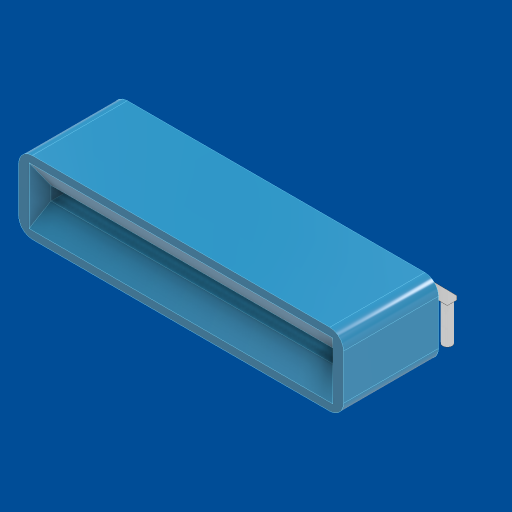
# Autodesk Inventor part: EEC12DRAN
Saved by Autodesk Inventor 2023.2 (Build 272271000, 271)
## iProperties
Created: 2023-01-27
Part Number: EEC12DRAN
Material: PBT Plastic
Document SubType Name: Modeling
Designer: agmlego
Density: 1.31 g/cm^3
Appearance: Sky Blue Dark
Mass: 4.18354 g
Surface Area: 30.0335 cm^2
Volume: 3.19354 cm^3
Author: agmlego
Autodesk Inventor part; units mm, degrees
ref_plane "YZ Plane" through (0, 0, 0) normal (1, 0, 0) x (0, 1, 0)
ref_plane "XZ Plane" through (0, 0, 0) normal (0, 1, 0) x (-1, 0, 0)
sketch "Sketch1" plane through (0, 0, 0) normal (0, 0, 1) x (1, 0, 0)
  line L0 (-18.7325, 4.191) -> (18.7325, 4.191)
  line L1 (18.7325, 4.191) -> (18.7325, -4.191)
  line L2 (18.7325, -4.191) -> (-18.7325, -4.191)
  line L3 (-18.7325, -4.191) -> (-18.7325, 4.191)
  line L4 (0, 4.191) -> (0, -4.191) construction
  point P0 (0, 0)
  point P1 (0, 0)
  dimension "dim_f" = 8.382
  dimension "dim_c" = 37.465
  constraints: 10 end point, 3 midpoint, 2 parallel, 1 coincident, 1 horizontal, 1 perpendicular
  measures "dim_f" distance of L2.end L0.start
  measures "dim_c" distance of L1.end L2.end
extrude "Extrusion1" add sketch "Sketch1" against normal blind 10.95
sketch "Sketch2" plane through (0, 0, 0) normal (0, 0, 1) x (1, 0, 0)
  line L0 (-16.51, 0.7874) -> (16.51, 0.7874)
  line L1 (16.51, 0.7874) -> (16.51, -0.7874)
  line L2 (16.51, -0.7874) -> (-16.51, -0.7874)
  line L3 (-16.51, -0.7874) -> (-16.51, 0.7874)
  line L4 (0, 0.7874) -> (0, -0.7874) construction
  point P0 (0, 0)
  point P1 (0, 0)
  dimension "dim_b" = 33.02
  dimension "card_width" = 1.5748
  constraints: 10 end point, 3 midpoint, 2 parallel, 1 coincident, 1 horizontal, 1 perpendicular
  measures "dim_b" distance of L0.start L0.end
  measures "card_width" distance of L2.end L0.start
extrude "Extrusion2" cut sketch "Sketch2" against normal blind 6.731
chamfer "Chamfer1" distance 2.5 distance2 1.5 2 edges at (0, 0.7874, 0) (0, -0.7874, 0) measured on face at (-5.5033, 3.0565, 0)
chamfer "Chamfer2" distance 1 distance2 1.5 2 edges at (-16.51, 0, 0) (16.51, 0, 0) measured on face at (-5.5033, 3.8898, 0)
fillet "Fillet1" radius 1.5875 4 edges at (-18.7325, 4.191, -5.475) (-18.7325, -4.191, -5.475) (18.7325, -4.191, -5.475) (18.7325, 4.191, -5.475)
sketch "Sketch3" plane through (0, 0, -10.95) normal (0, 0, -1) x (-1, 0, 0)
  line L0 (-14.5161, 2.5273) -> (-13.4239, 2.5273)
  line L1 (-13.4239, 2.5273) -> (-13.4239, 1.4351)
  line L2 (-13.4239, 1.4351) -> (-14.5161, 1.4351)
  line L3 (-14.5161, 1.4351) -> (-14.5161, 2.5273)
  line L4 (-11.9761, 2.5273) -> (-10.8839, 2.5273)
  line L5 (-10.8839, 2.5273) -> (-10.8839, 1.4351)
  line L6 (-10.8839, 1.4351) -> (-11.9761, 1.4351)
  line L7 (-11.9761, 1.4351) -> (-11.9761, 2.5273)
  line L8 (-9.4361, 2.5273) -> (-8.3439, 2.5273)
  line L9 (-8.3439, 2.5273) -> (-8.3439, 1.4351)
  line L10 (-8.3439, 1.4351) -> (-9.4361, 1.4351)
  line L11 (-9.4361, 1.4351) -> (-9.4361, 2.5273)
  line L12 (-6.8961, 2.5273) -> (-5.8039, 2.5273)
  line L13 (-5.8039, 2.5273) -> (-5.8039, 1.4351)
  line L14 (-5.8039, 1.4351) -> (-6.8961, 1.4351)
  line L15 (-6.8961, 1.4351) -> (-6.8961, 2.5273)
  line L16 (-4.3561, 2.5273) -> (-3.2639, 2.5273)
  line L17 (-3.2639, 2.5273) -> (-3.2639, 1.4351)
  line L18 (-3.2639, 1.4351) -> (-4.3561, 1.4351)
  line L19 (-4.3561, 1.4351) -> (-4.3561, 2.5273)
  line L20 (-1.8161, 2.5273) -> (-0.7239, 2.5273)
  line L21 (-0.7239, 2.5273) -> (-0.7239, 1.4351)
  line L22 (-0.7239, 1.4351) -> (-1.8161, 1.4351)
  line L23 (-1.8161, 1.4351) -> (-1.8161, 2.5273)
  line L24 (0.7239, 2.5273) -> (1.8161, 2.5273)
  line L25 (1.8161, 2.5273) -> (1.8161, 1.4351)
  line L26 (1.8161, 1.4351) -> (0.7239, 1.4351)
  line L27 (0.7239, 1.4351) -> (0.7239, 2.5273)
  line L28 (3.2639, 2.5273) -> (4.3561, 2.5273)
  line L29 (4.3561, 2.5273) -> (4.3561, 1.4351)
  line L30 (4.3561, 1.4351) -> (3.2639, 1.4351)
  line L31 (3.2639, 1.4351) -> (3.2639, 2.5273)
  line L32 (5.8039, 2.5273) -> (6.8961, 2.5273)
  line L33 (6.8961, 2.5273) -> (6.8961, 1.4351)
  line L34 (6.8961, 1.4351) -> (5.8039, 1.4351)
  line L35 (5.8039, 1.4351) -> (5.8039, 2.5273)
  line L36 (8.3439, 2.5273) -> (9.4361, 2.5273)
  line L37 (9.4361, 2.5273) -> (9.4361, 1.4351)
  line L38 (9.4361, 1.4351) -> (8.3439, 1.4351)
  line L39 (8.3439, 1.4351) -> (8.3439, 2.5273)
  line L40 (10.8839, 2.5273) -> (11.9761, 2.5273)
  line L41 (11.9761, 2.5273) -> (11.9761, 1.4351)
  line L42 (11.9761, 1.4351) -> (10.8839, 1.4351)
  line L43 (10.8839, 1.4351) -> (10.8839, 2.5273)
  line L44 (13.4239, 2.5273) -> (14.5161, 2.5273)
  line L45 (14.5161, 2.5273) -> (14.5161, 1.4351)
  line L46 (14.5161, 1.4351) -> (13.4239, 1.4351)
  line L47 (13.4239, 1.4351) -> (13.4239, 2.5273)
  line L48 (-14.5161, -1.4351) -> (-13.4239, -1.4351)
  line L49 (-13.4239, -1.4351) -> (-13.4239, -2.5273)
  line L50 (-13.4239, -2.5273) -> (-14.5161, -2.5273)
  line L51 (-14.5161, -2.5273) -> (-14.5161, -1.4351)
  line L52 (-11.9761, -1.4351) -> (-10.8839, -1.4351)
  line L53 (-10.8839, -1.4351) -> (-10.8839, -2.5273)
  line L54 (-10.8839, -2.5273) -> (-11.9761, -2.5273)
  line L55 (-11.9761, -2.5273) -> (-11.9761, -1.4351)
  line L56 (-9.4361, -1.4351) -> (-8.3439, -1.4351)
  line L57 (-8.3439, -1.4351) -> (-8.3439, -2.5273)
  line L58 (-8.3439, -2.5273) -> (-9.4361, -2.5273)
  line L59 (-9.4361, -2.5273) -> (-9.4361, -1.4351)
  line L60 (-6.8961, -1.4351) -> (-5.8039, -1.4351)
  line L61 (-5.8039, -1.4351) -> (-5.8039, -2.5273)
  line L62 (-5.8039, -2.5273) -> (-6.8961, -2.5273)
  line L63 (-6.8961, -2.5273) -> (-6.8961, -1.4351)
  line L64 (-4.3561, -1.4351) -> (-3.2639, -1.4351)
  line L65 (-3.2639, -1.4351) -> (-3.2639, -2.5273)
  line L66 (-3.2639, -2.5273) -> (-4.3561, -2.5273)
  line L67 (-4.3561, -2.5273) -> (-4.3561, -1.4351)
  line L68 (-1.8161, -1.4351) -> (-0.7239, -1.4351)
  line L69 (-0.7239, -1.4351) -> (-0.7239, -2.5273)
  line L70 (-0.7239, -2.5273) -> (-1.8161, -2.5273)
  line L71 (-1.8161, -2.5273) -> (-1.8161, -1.4351)
  line L72 (0.7239, -1.4351) -> (1.8161, -1.4351)
  line L73 (1.8161, -1.4351) -> (1.8161, -2.5273)
  line L74 (1.8161, -2.5273) -> (0.7239, -2.5273)
  line L75 (0.7239, -2.5273) -> (0.7239, -1.4351)
  line L76 (3.2639, -1.4351) -> (4.3561, -1.4351)
  line L77 (4.3561, -1.4351) -> (4.3561, -2.5273)
  line L78 (4.3561, -2.5273) -> (3.2639, -2.5273)
  line L79 (3.2639, -2.5273) -> (3.2639, -1.4351)
  line L80 (5.8039, -1.4351) -> (6.8961, -1.4351)
  line L81 (6.8961, -1.4351) -> (6.8961, -2.5273)
  line L82 (6.8961, -2.5273) -> (5.8039, -2.5273)
  line L83 (5.8039, -2.5273) -> (5.8039, -1.4351)
  line L84 (8.3439, -1.4351) -> (9.4361, -1.4351)
  line L85 (9.4361, -1.4351) -> (9.4361, -2.5273)
  line L86 (9.4361, -2.5273) -> (8.3439, -2.5273)
  line L87 (8.3439, -2.5273) -> (8.3439, -1.4351)
  line L88 (10.8839, -1.4351) -> (11.9761, -1.4351)
  line L89 (11.9761, -1.4351) -> (11.9761, -2.5273)
  line L90 (11.9761, -2.5273) -> (10.8839, -2.5273)
  line L91 (10.8839, -2.5273) -> (10.8839, -1.4351)
  line L92 (13.4239, -1.4351) -> (14.5161, -1.4351)
  line L93 (14.5161, -1.4351) -> (14.5161, -2.5273)
  line L94 (14.5161, -2.5273) -> (13.4239, -2.5273)
  line L95 (13.4239, -2.5273) -> (13.4239, -1.4351)
  line L96 (-0.7239, 1.4351) -> (0.7239, -1.4351) construction
  point P0 (0, 0)
  point P1 (0, 0)
  dimension "pin_pitch" = 2.54
  dimension "row_pitch" = 3.9624
  dimension "pin_dia" = 1.0922
  constraints: 194 end point, 2 collinear, 2 horizontal, 2 parallel, 2 perpendicular, 1 coincident, 1 midpoint, 1 vertical, 182 other
  measures "pin_pitch" distance of L0.start L4.start
  measures "row_pitch" distance of L0.start L48.start
  measures "pin_dia" distance of L0.start L0.end
ref_plane "Work Plane2" through (-17.145, -7.366, 0) normal (0, -1, 0) x (1, 0, 0)
sketch "Sketch4" plane through (-17.145, -7.366, 0) normal (0, -1, 0) x (1, 0, 0)
  line L0 (35.8775, -10.95) -> (34.29, -10.95) construction
  line L1 (34.29, -10.95) -> (35.8775, -10.95) construction
  line L2 (34.29, -10.95) -> (0, -10.95) construction
  line L3 (-1.5875, -10.95) -> (0, -10.95) construction
  line L4 (0, -10.95) -> (-1.5875, -10.95) construction
  line L5 (0, -10.95) -> (34.29, -10.95) construction
  line L6 (31.6611, -12.22) -> (30.5689, -12.22)
  line L7 (30.5689, -12.22) -> (30.5689, -13.3122)
  line L8 (30.5689, -13.3122) -> (31.6611, -13.3122)
  line L9 (31.6611, -13.3122) -> (31.6611, -12.22)
  line L10 (29.1211, -12.22) -> (28.0289, -12.22)
  line L11 (28.0289, -12.22) -> (28.0289, -13.3122)
  line L12 (28.0289, -13.3122) -> (29.1211, -13.3122)
  line L13 (29.1211, -13.3122) -> (29.1211, -12.22)
  line L14 (26.5811, -12.22) -> (25.4889, -12.22)
  line L15 (25.4889, -12.22) -> (25.4889, -13.3122)
  line L16 (25.4889, -13.3122) -> (26.5811, -13.3122)
  line L17 (26.5811, -13.3122) -> (26.5811, -12.22)
  line L18 (24.0411, -12.22) -> (22.9489, -12.22)
  line L19 (22.9489, -12.22) -> (22.9489, -13.3122)
  line L20 (22.9489, -13.3122) -> (24.0411, -13.3122)
  line L21 (24.0411, -13.3122) -> (24.0411, -12.22)
  line L22 (21.5011, -12.22) -> (20.4089, -12.22)
  line L23 (20.4089, -12.22) -> (20.4089, -13.3122)
  line L24 (20.4089, -13.3122) -> (21.5011, -13.3122)
  line L25 (21.5011, -13.3122) -> (21.5011, -12.22)
  line L26 (18.9611, -12.22) -> (17.8689, -12.22)
  line L27 (17.8689, -12.22) -> (17.8689, -13.3122)
  line L28 (17.8689, -13.3122) -> (18.9611, -13.3122)
  line L29 (18.9611, -13.3122) -> (18.9611, -12.22)
  line L30 (16.4211, -12.22) -> (15.3289, -12.22)
  line L31 (15.3289, -12.22) -> (15.3289, -13.3122)
  line L32 (15.3289, -13.3122) -> (16.4211, -13.3122)
  line L33 (16.4211, -13.3122) -> (16.4211, -12.22)
  line L34 (13.8811, -12.22) -> (12.7889, -12.22)
  line L35 (12.7889, -12.22) -> (12.7889, -13.3122)
  line L36 (12.7889, -13.3122) -> (13.8811, -13.3122)
  line L37 (13.8811, -13.3122) -> (13.8811, -12.22)
  line L38 (11.3411, -12.22) -> (10.2489, -12.22)
  line L39 (10.2489, -12.22) -> (10.2489, -13.3122)
  line L40 (10.2489, -13.3122) -> (11.3411, -13.3122)
  line L41 (11.3411, -13.3122) -> (11.3411, -12.22)
  line L42 (8.8011, -12.22) -> (7.7089, -12.22)
  line L43 (7.7089, -12.22) -> (7.7089, -13.3122)
  line L44 (7.7089, -13.3122) -> (8.8011, -13.3122)
  line L45 (8.8011, -13.3122) -> (8.8011, -12.22)
  line L46 (6.2611, -12.22) -> (5.1689, -12.22)
  line L47 (5.1689, -12.22) -> (5.1689, -13.3122)
  line L48 (5.1689, -13.3122) -> (6.2611, -13.3122)
  line L49 (6.2611, -13.3122) -> (6.2611, -12.22)
  line L50 (3.7211, -12.22) -> (2.6289, -12.22)
  line L51 (2.6289, -12.22) -> (2.6289, -13.3122)
  line L52 (2.6289, -13.3122) -> (3.7211, -13.3122)
  line L53 (3.7211, -13.3122) -> (3.7211, -12.22)
  line L54 (31.6611, -16.1824) -> (30.5689, -16.1824)
  line L55 (30.5689, -16.1824) -> (30.5689, -17.2746)
  line L56 (30.5689, -17.2746) -> (31.6611, -17.2746)
  line L57 (31.6611, -17.2746) -> (31.6611, -16.1824)
  line L58 (29.1211, -16.1824) -> (28.0289, -16.1824)
  line L59 (28.0289, -16.1824) -> (28.0289, -17.2746)
  line L60 (28.0289, -17.2746) -> (29.1211, -17.2746)
  line L61 (29.1211, -17.2746) -> (29.1211, -16.1824)
  line L62 (26.5811, -16.1824) -> (25.4889, -16.1824)
  line L63 (25.4889, -16.1824) -> (25.4889, -17.2746)
  line L64 (25.4889, -17.2746) -> (26.5811, -17.2746)
  line L65 (26.5811, -17.2746) -> (26.5811, -16.1824)
  line L66 (24.0411, -16.1824) -> (22.9489, -16.1824)
  line L67 (22.9489, -16.1824) -> (22.9489, -17.2746)
  line L68 (22.9489, -17.2746) -> (24.0411, -17.2746)
  line L69 (24.0411, -17.2746) -> (24.0411, -16.1824)
  line L70 (21.5011, -16.1824) -> (20.4089, -16.1824)
  line L71 (20.4089, -16.1824) -> (20.4089, -17.2746)
  line L72 (20.4089, -17.2746) -> (21.5011, -17.2746)
  line L73 (21.5011, -17.2746) -> (21.5011, -16.1824)
  line L74 (18.9611, -16.1824) -> (17.8689, -16.1824)
  line L75 (17.8689, -16.1824) -> (17.8689, -17.2746)
  line L76 (17.8689, -17.2746) -> (18.9611, -17.2746)
  line L77 (18.9611, -17.2746) -> (18.9611, -16.1824)
  line L78 (16.4211, -16.1824) -> (15.3289, -16.1824)
  line L79 (15.3289, -16.1824) -> (15.3289, -17.2746)
  line L80 (15.3289, -17.2746) -> (16.4211, -17.2746)
  line L81 (16.4211, -17.2746) -> (16.4211, -16.1824)
  line L82 (13.8811, -16.1824) -> (12.7889, -16.1824)
  line L83 (12.7889, -16.1824) -> (12.7889, -17.2746)
  line L84 (12.7889, -17.2746) -> (13.8811, -17.2746)
  line L85 (13.8811, -17.2746) -> (13.8811, -16.1824)
  line L86 (11.3411, -16.1824) -> (10.2489, -16.1824)
  line L87 (10.2489, -16.1824) -> (10.2489, -17.2746)
  line L88 (10.2489, -17.2746) -> (11.3411, -17.2746)
  line L89 (11.3411, -17.2746) -> (11.3411, -16.1824)
  line L90 (8.8011, -16.1824) -> (7.7089, -16.1824)
  line L91 (7.7089, -16.1824) -> (7.7089, -17.2746)
  line L92 (7.7089, -17.2746) -> (8.8011, -17.2746)
  line L93 (8.8011, -17.2746) -> (8.8011, -16.1824)
  line L94 (6.2611, -16.1824) -> (5.1689, -16.1824)
  line L95 (5.1689, -16.1824) -> (5.1689, -17.2746)
  line L96 (5.1689, -17.2746) -> (6.2611, -17.2746)
  line L97 (6.2611, -17.2746) -> (6.2611, -16.1824)
  line L98 (3.7211, -16.1824) -> (2.6289, -16.1824)
  line L99 (2.6289, -16.1824) -> (2.6289, -17.2746)
  line L100 (2.6289, -17.2746) -> (3.7211, -17.2746)
  line L101 (3.7211, -17.2746) -> (3.7211, -16.1824)
  point P0 (17.145, 0)
  point P1 (31.6611, -10.95)
  point P2 (31.6611, -10.95)
  point P3 (31.6611, -10.95)
  point P4 (30.5689, -10.95)
  point P5 (30.5689, -10.95)
  point P6 (30.5689, -10.95)
  point P7 (28.0289, -10.95)
  point P8 (29.1211, -10.95)
  point P9 (25.4889, -10.95)
  point P10 (26.5811, -10.95)
  point P11 (22.9489, -10.95)
  point P12 (24.0411, -10.95)
  point P13 (20.4089, -10.95)
  point P14 (21.5011, -10.95)
  point P15 (17.8689, -10.95)
  point P16 (18.9611, -10.95)
  point P17 (15.3289, -10.95)
  point P18 (16.4211, -10.95)
  point P19 (12.7889, -10.95)
  point P20 (13.8811, -10.95)
  point P21 (10.2489, -10.95)
  point P22 (11.3411, -10.95)
  point P23 (7.7089, -10.95)
  point P24 (8.8011, -10.95)
  point P25 (5.1689, -10.95)
  point P26 (6.2611, -10.95)
  point P27 (2.6289, -10.95)
  point P28 (3.7211, -10.95)
  point P29 (30.5689, -14.9124)
  point P30 (31.6611, -14.9124)
  point P31 (28.0289, -14.9124)
  point P32 (29.1211, -14.9124)
  point P33 (25.4889, -14.9124)
  point P34 (26.5811, -14.9124)
  point P35 (22.9489, -14.9124)
  point P36 (24.0411, -14.9124)
  point P37 (20.4089, -14.9124)
  point P38 (21.5011, -14.9124)
  point P39 (17.8689, -14.9124)
  point P40 (18.9611, -14.9124)
  point P41 (15.3289, -14.9124)
  point P42 (16.4211, -14.9124)
  point P43 (12.7889, -14.9124)
  point P44 (13.8811, -14.9124)
  point P45 (10.2489, -14.9124)
  point P46 (11.3411, -14.9124)
  point P47 (7.7089, -14.9124)
  point P48 (8.8011, -14.9124)
  point P49 (5.1689, -14.9124)
  point P50 (6.2611, -14.9124)
  point P51 (2.6289, -14.9124)
  point P52 (3.7211, -14.9124)
  dimension "pin_offset" = 1.27
  dimension "d29" = 2.54
  dimension "d32" = 3.9624
  constraints: 192 end point, 48 point on line, 2 collinear, 2 horizontal, 2 parallel, 2 perpendicular, 1 vertical, 228 other
  measures "pin_offset" distance between parallel lines of L6 L2
  measures "d29" distance of L7.end L11.end
  measures "d32" distance of L7.end L55.end
sketch "Sketch5" plane through (0, 0, 0) normal (1, 0, 0) x (0, 1, 0)
  line L0 (2.5273, -10.95) -> (2.5273, -12.22)
  line L1 (2.5273, -12.22) -> (-2.6035, -17.2746)
  line L2 (-2.6035, -17.2746) -> (-7.366, -17.2746)
  line L3 (-1.4351, -10.95) -> (-1.4351, -12.22)
  line L4 (-1.4351, -12.22) -> (-2.5438, -13.3122)
  line L5 (-2.5438, -13.3122) -> (-7.366, -13.3122)
  point P0 (0, 0)
  dimension "d35" = 4.7625
  dimension "d36" = 1.27
  constraints: 12 end point, 2 parallel, 2 perpendicular, 2 vertical
  measures "d35" distance of L1.end L2.end
  measures "d36" distance of L0.start L0.end
sweep "Sweep1" add profiles "Sketch3" path "Sketch5" separate body path curves L0 L1 L2 contours L0 L1 L2 L3 | L4 L5 L6 L7 | L8 L9 L10 L11 | L12 L13 L14 L15 | L16 L17 L18 L19 | L20 L21 L22 L23 | L24 L25 L26 L27 | L28 L29 L30 L31 | L32 L33 L34 L35 | L36 L37 L38 L39 | L40 L41 L42 L43 | L44 L45 L46 L47
sweep "Sweep2" add profiles "Sketch3" path "Sketch5" separate body path curves L3 L4 L5 contours L48 L49 L50 L51 | L52 L53 L54 L55 | L56 L57 L58 L59 | L60 L61 L62 L63 | L64 L65 L66 L67 | L68 L69 L70 L71 | L72 L73 L74 L75 | L76 L77 L78 L79 | L80 L81 L82 L83 | L84 L85 L86 L87 | L88 L89 L90 L91 | L92 L93 L94 L95
sketch "Sketch6" plane through (13.4239, -7.366, -16.1824) normal (0, -1, 0) x (1, 0, 0)
  circle A0 centre (0.5461, -0.5461) radius 0.5461
  line L0 (-7.62, -1.0922) -> (-6.5278, -1.0922) projected
  line L1 (-5.08, -1.0922) -> (-3.9878, -1.0922) projected
  line L2 (-5.08, 0) -> (-5.08, -1.0922) projected
  line L3 (-3.9878, -1.0922) -> (-3.9878, 0) projected
  line L4 (-2.54, 0) -> (-2.54, -1.0922) projected
  line L5 (-7.62, 0) -> (-7.62, -1.0922) projected
  line L6 (-6.5278, 0) -> (-7.62, 0) projected
  line L7 (-3.9878, 0) -> (-5.08, 0) projected
  line L8 (-3.9878, 0) -> (-5.08, 0) projected
  line L9 (-6.5278, -1.0922) -> (-6.5278, 0) projected
  line L10 (-6.5278, 0) -> (-7.62, 0) projected
  line L11 (-10.16, 0) -> (-10.16, -1.0922) projected
  line L12 (-9.0678, -1.0922) -> (-9.0678, 0) projected
  line L13 (-1.4478, -1.0922) -> (-1.4478, 0) projected
  line L14 (-1.4478, 0) -> (-2.54, 0) projected
  line L15 (-1.4478, 0) -> (-2.54, 0) projected
  line L16 (-2.54, -1.0922) -> (-1.4478, -1.0922) projected
  line L17 (-2.54, -1.0922) -> (-1.4478, -1.0922) projected
  line L18 (-7.62, -1.0922) -> (-6.5278, -1.0922) projected
  line L19 (-9.0678, 0) -> (-10.16, 0) projected
  line L20 (-10.16, -1.0922) -> (-9.0678, -1.0922) projected
  line L21 (-10.16, -1.0922) -> (-9.0678, -1.0922) projected
  line L22 (-9.0678, 0) -> (-10.16, 0) projected
  line L23 (-14.1478, 0) -> (-15.24, 0) projected
  line L24 (-14.1478, -1.0922) -> (-14.1478, 0) projected
  line L25 (-15.24, -1.0922) -> (-14.1478, -1.0922) projected
  line L26 (-11.6078, 0) -> (-12.7, 0) projected
  line L27 (-15.24, 0) -> (-15.24, -1.0922) projected
  line L28 (-11.6078, 0) -> (-12.7, 0) projected
  line L29 (-12.7, -1.0922) -> (-11.6078, -1.0922) projected
  line L30 (-20.32, 0) -> (-20.32, -1.0922) projected
  line L31 (-19.2278, -1.0922) -> (-19.2278, 0) projected
  line L32 (-19.2278, 0) -> (-20.32, 0) projected
  line L33 (-19.2278, 0) -> (-20.32, 0) projected
  line L34 (-20.32, -1.0922) -> (-19.2278, -1.0922) projected
  line L35 (-20.32, -1.0922) -> (-19.2278, -1.0922) projected
  line L36 (-17.78, 0) -> (-17.78, -1.0922) projected
  line L37 (-16.6878, -1.0922) -> (-16.6878, 0) projected
  line L38 (-14.1478, 0) -> (-15.24, 0) projected
  line L39 (-15.24, -1.0922) -> (-14.1478, -1.0922) projected
  line L40 (-17.78, -1.0922) -> (-16.6878, -1.0922) projected
  line L41 (-11.6078, -1.0922) -> (-11.6078, 0) projected
  line L42 (-12.7, 0) -> (-12.7, -1.0922) projected
  line L43 (-17.78, -1.0922) -> (-16.6878, -1.0922) projected
  line L44 (-16.6878, 0) -> (-17.78, 0) projected
  line L45 (-12.7, -1.0922) -> (-11.6078, -1.0922) projected
  line L46 (-26.8478, -1.0922) -> (-26.8478, 0) projected
  line L47 (-27.94, 0) -> (-27.94, -1.0922) projected
  line L48 (-26.8478, 0) -> (-27.94, 0) projected
  line L49 (-27.94, -1.0922) -> (-26.8478, -1.0922) projected
  line L50 (-26.8478, 0) -> (-27.94, 0) projected
  line L51 (-27.94, -1.0922) -> (-26.8478, -1.0922) projected
  line L52 (-22.86, 0) -> (-22.86, -1.0922) projected
  line L53 (-21.7678, -1.0922) -> (-21.7678, 0) projected
  line L54 (-22.86, -1.0922) -> (-21.7678, -1.0922) projected
  line L55 (-21.7678, 0) -> (-22.86, 0) projected
  line L56 (-21.7678, 0) -> (-22.86, 0) projected
  line L57 (-22.86, -1.0922) -> (-21.7678, -1.0922) projected
  line L58 (-25.4, -1.0922) -> (-24.3078, -1.0922) projected
  line L59 (-25.4, 0) -> (-25.4, -1.0922) projected
  line L60 (-24.3078, -1.0922) -> (-24.3078, 0) projected
  line L61 (-24.3078, 0) -> (-25.4, 0) projected
  line L62 (-24.3078, 0) -> (-25.4, 0) projected
  line L63 (-25.4, -1.0922) -> (-24.3078, -1.0922) projected
  line L64 (-16.6878, 0) -> (-17.78, 0) projected
  line L65 (0, 0) -> (0, -1.0922) projected
  line L66 (1.0922, -1.0922) -> (1.0922, 0) projected
  line L67 (1.0922, 0) -> (0, 0) projected
  line L68 (0, -1.0922) -> (1.0922, -1.0922) projected
  line L69 (1.0922, 0) -> (0, 0) projected
  line L70 (0, -1.0922) -> (1.0922, -1.0922) projected
  line L71 (-5.08, -1.0922) -> (-3.9878, -1.0922) projected
  line L72 (-17.78, 3.9624) -> (-16.6878, 3.9624) projected
  line L73 (-20.32, 3.9624) -> (-19.2278, 3.9624) projected
  line L74 (-12.7, 3.9624) -> (-11.6078, 3.9624) projected
  line L75 (-15.24, 3.9624) -> (-14.1478, 3.9624) projected
  line L76 (-27.94, 3.9624) -> (-26.8478, 3.9624) projected
  line L77 (-22.86, 3.9624) -> (-21.7678, 3.9624) projected
  line L78 (-25.4, 3.9624) -> (-24.3078, 3.9624) projected
  line L79 (-10.16, 3.9624) -> (-9.0678, 3.9624) projected
  line L80 (0, 3.9624) -> (1.0922, 3.9624) projected
  line L81 (-7.62, 3.9624) -> (-6.5278, 3.9624) projected
  line L82 (-5.08, 3.9624) -> (-3.9878, 3.9624) projected
  line L83 (-2.54, 3.9624) -> (-1.4478, 3.9624) projected
  line L84 (-20.32, 3.9624) -> (-19.2278, 3.9624) projected
  line L85 (-19.2278, 3.9624) -> (-20.32, 3.9624) projected
  line L86 (-19.2278, 3.9624) -> (-19.2278, 2.8702) projected
  line L87 (-20.32, 3.9624) -> (-20.32, 2.8702) projected
  line L88 (-20.32, 2.8702) -> (-19.2278, 2.8702) projected
  line L89 (-19.2278, 3.9624) -> (-20.32, 3.9624) projected
  line L90 (-19.2278, 2.8702) -> (-19.2278, 3.9624) projected
  line L91 (-20.32, 2.8702) -> (-19.2278, 2.8702) projected
  line L92 (-20.32, 3.9624) -> (-20.32, 2.8702) projected
  line L93 (-25.4, 3.9624) -> (-25.4, 2.8702) projected
  line L94 (-24.3078, 3.9624) -> (-25.4, 3.9624) projected
  line L95 (-25.4, 3.9624) -> (-24.3078, 3.9624) projected
  line L96 (-24.3078, 3.9624) -> (-24.3078, 2.8702) projected
  line L97 (-25.4, 2.8702) -> (-24.3078, 2.8702) projected
  line L98 (-15.24, 3.9624) -> (-15.24, 2.8702) projected
  line L99 (-14.1478, 3.9624) -> (-15.24, 3.9624) projected
  line L100 (-15.24, 3.9624) -> (-14.1478, 3.9624) projected
  line L101 (-14.1478, 3.9624) -> (-14.1478, 2.8702) projected
  line L102 (-15.24, 2.8702) -> (-14.1478, 2.8702) projected
  line L103 (-16.6878, 3.9624) -> (-16.6878, 2.8702) projected
  line L104 (-17.78, 3.9624) -> (-17.78, 2.8702) projected
  line L105 (-17.78, 2.8702) -> (-16.6878, 2.8702) projected
  line L106 (-16.6878, 3.9624) -> (-17.78, 3.9624) projected
  line L107 (-17.78, 3.9624) -> (-16.6878, 3.9624) projected
  line L108 (-17.78, 3.9624) -> (-17.78, 2.8702) projected
  line L109 (-16.6878, 2.8702) -> (-16.6878, 3.9624) projected
  line L110 (-16.6878, 3.9624) -> (-17.78, 3.9624) projected
  line L111 (-17.78, 2.8702) -> (-16.6878, 2.8702) projected
  line L112 (-15.24, 3.9624) -> (-15.24, 2.8702) projected
  line L113 (-14.1478, 2.8702) -> (-14.1478, 3.9624) projected
  line L114 (-14.1478, 3.9624) -> (-15.24, 3.9624) projected
  line L115 (-15.24, 2.8702) -> (-14.1478, 2.8702) projected
  line L116 (-22.86, 3.9624) -> (-22.86, 2.8702) projected
  line L117 (-21.7678, 2.8702) -> (-21.7678, 3.9624) projected
  line L118 (-21.7678, 3.9624) -> (-22.86, 3.9624) projected
  line L119 (-22.86, 2.8702) -> (-21.7678, 2.8702) projected
  line L120 (-22.86, 3.9624) -> (-22.86, 2.8702) projected
  line L121 (-21.7678, 3.9624) -> (-21.7678, 2.8702) projected
  line L122 (-22.86, 3.9624) -> (-21.7678, 3.9624) projected
  line L123 (-21.7678, 3.9624) -> (-22.86, 3.9624) projected
  line L124 (-22.86, 2.8702) -> (-21.7678, 2.8702) projected
  line L125 (-26.8478, 3.9624) -> (-26.8478, 2.8702) projected
  line L126 (-27.94, 3.9624) -> (-27.94, 2.8702) projected
  line L127 (-27.94, 2.8702) -> (-26.8478, 2.8702) projected
  line L128 (-26.8478, 3.9624) -> (-27.94, 3.9624) projected
  line L129 (-27.94, 3.9624) -> (-26.8478, 3.9624) projected
  line L130 (-27.94, 3.9624) -> (-27.94, 2.8702) projected
  line L131 (-26.8478, 2.8702) -> (-26.8478, 3.9624) projected
  line L132 (-26.8478, 3.9624) -> (-27.94, 3.9624) projected
  line L133 (-27.94, 2.8702) -> (-26.8478, 2.8702) projected
  line L134 (-25.4, 3.9624) -> (-25.4, 2.8702) projected
  line L135 (-24.3078, 3.9624) -> (-25.4, 3.9624) projected
  line L136 (-25.4, 2.8702) -> (-24.3078, 2.8702) projected
  line L137 (-24.3078, 2.8702) -> (-24.3078, 3.9624) projected
  line L138 (-9.0678, 3.9624) -> (-10.16, 3.9624) projected
  line L139 (-9.0678, 3.9624) -> (-9.0678, 2.8702) projected
  line L140 (-10.16, 3.9624) -> (-10.16, 2.8702) projected
  line L141 (-10.16, 2.8702) -> (-9.0678, 2.8702) projected
  line L142 (-9.0678, 3.9624) -> (-10.16, 3.9624) projected
  line L143 (-10.16, 3.9624) -> (-10.16, 2.8702) projected
  line L144 (-10.16, 2.8702) -> (-9.0678, 2.8702) projected
  line L145 (-9.0678, 2.8702) -> (-9.0678, 3.9624) projected
  line L146 (-10.16, 3.9624) -> (-9.0678, 3.9624) projected
  line L147 (-6.5278, 3.9624) -> (-7.62, 3.9624) projected
  line L148 (-7.62, 2.8702) -> (-6.5278, 2.8702) projected
  line L149 (-7.62, 3.9624) -> (-6.5278, 3.9624) projected
  line L150 (-7.62, 3.9624) -> (-7.62, 2.8702) projected
  line L151 (-6.5278, 3.9624) -> (-6.5278, 2.8702) projected
  line L152 (-5.08, 3.9624) -> (-5.08, 2.8702) projected
  line L153 (-6.5278, 2.8702) -> (-6.5278, 3.9624) projected
  line L154 (-6.5278, 3.9624) -> (-7.62, 3.9624) projected
  line L155 (-7.62, 2.8702) -> (-6.5278, 2.8702) projected
  line L156 (-7.62, 3.9624) -> (-7.62, 2.8702) projected
  line L157 (-2.54, 3.9624) -> (-2.54, 2.8702) projected
  line L158 (-1.4478, 3.9624) -> (-1.4478, 2.8702) projected
  line L159 (-2.54, 2.8702) -> (-1.4478, 2.8702) projected
  line L160 (-3.9878, 3.9624) -> (-3.9878, 2.8702) projected
  line L161 (-3.9878, 3.9624) -> (-5.08, 3.9624) projected
  line L162 (-12.7, 3.9624) -> (-11.6078, 3.9624) projected
  line L163 (-11.6078, 3.9624) -> (-12.7, 3.9624) projected
  line L164 (-11.6078, 3.9624) -> (-11.6078, 2.8702) projected
  line L165 (-12.7, 3.9624) -> (-12.7, 2.8702) projected
  line L166 (-12.7, 2.8702) -> (-11.6078, 2.8702) projected
  line L167 (-11.6078, 3.9624) -> (-12.7, 3.9624) projected
  line L168 (-12.7, 3.9624) -> (-12.7, 2.8702) projected
  line L169 (-12.7, 2.8702) -> (-11.6078, 2.8702) projected
  line L170 (-11.6078, 2.8702) -> (-11.6078, 3.9624) projected
  line L171 (-5.08, 3.9624) -> (-3.9878, 3.9624) projected
  line L172 (-3.9878, 3.9624) -> (-5.08, 3.9624) projected
  line L173 (-5.08, 2.8702) -> (-3.9878, 2.8702) projected
  line L174 (-5.08, 2.8702) -> (-3.9878, 2.8702) projected
  line L175 (-2.54, 3.9624) -> (-1.4478, 3.9624) projected
  line L176 (-1.4478, 3.9624) -> (-2.54, 3.9624) projected
  line L177 (-2.54, 3.9624) -> (-2.54, 2.8702) projected
  line L178 (-1.4478, 2.8702) -> (-1.4478, 3.9624) projected
  line L179 (-1.4478, 3.9624) -> (-2.54, 3.9624) projected
  line L180 (-5.08, 3.9624) -> (-5.08, 2.8702) projected
  line L181 (-3.9878, 2.8702) -> (-3.9878, 3.9624) projected
  line L182 (-2.54, 2.8702) -> (-1.4478, 2.8702) projected
  line L183 (0, 3.9624) -> (1.0922, 3.9624) projected
  line L184 (1.0922, 3.9624) -> (0, 3.9624) projected
  line L185 (0, 3.9624) -> (0, 2.8702) projected
  line L186 (1.0922, 3.9624) -> (1.0922, 2.8702) projected
  line L187 (0, 2.8702) -> (1.0922, 2.8702) projected
  line L188 (1.0922, 3.9624) -> (0, 3.9624) projected
  line L189 (0, 3.9624) -> (0, 2.8702) projected
  line L190 (0, 2.8702) -> (1.0922, 2.8702) projected
  line L191 (1.0922, 2.8702) -> (1.0922, 3.9624) projected
  circle A1 centre (-1.9939, -0.5461) radius 0.5461
  circle A2 centre (-4.5339, -0.5461) radius 0.5461
  circle A3 centre (-7.0739, -0.5461) radius 0.5461
  circle A4 centre (-9.6139, -0.5461) radius 0.5461
  circle A5 centre (-12.1539, -0.5461) radius 0.5461
  circle A6 centre (-14.6939, -0.5461) radius 0.5461
  circle A7 centre (-17.2339, -0.5461) radius 0.5461
  circle A8 centre (-19.7739, -0.5461) radius 0.5461
  circle A9 centre (-22.3139, -0.5461) radius 0.5461
  circle A10 centre (-24.8539, -0.5461) radius 0.5461
  circle A11 centre (-27.3939, -0.5461) radius 0.5461
  circle A12 centre (0.5461, 3.4163) radius 0.5461
  circle A13 centre (-1.9939, 3.4163) radius 0.5461
  circle A14 centre (-4.5339, 3.4163) radius 0.5461
  circle A15 centre (-7.0739, 3.4163) radius 0.5461
  circle A16 centre (-9.6139, 3.4163) radius 0.5461
  circle A17 centre (-12.1539, 3.4163) radius 0.5461
  circle A18 centre (-14.6939, 3.4163) radius 0.5461
  circle A19 centre (-17.2339, 3.4163) radius 0.5461
  circle A20 centre (-19.7739, 3.4163) radius 0.5461
  circle A21 centre (-22.3139, 3.4163) radius 0.5461
  circle A22 centre (-24.8539, 3.4163) radius 0.5461
  circle A23 centre (-27.3939, 3.4163) radius 0.5461
  point P0 (-13.4239, 16.1824)
  point P1 (0.5461, 0)
  point P2 (0, -0.5461)
  point P3 (1.0922, -0.5461)
  point P4 (0.5461, -1.0922)
  dimension "d41" = 1.0922
  dimension "d44" = 2.54
  dimension "d47" = 3.9624
  constraints: 24 centre point, 2 tangent, 1 horizontal, 1 vertical, 46 other
  measures "d41" diameter of A0
  measures "d44" distance of A0.centre A1.centre
  measures "d47" distance of A0.centre A12.centre
extrude "Extrusion3" cut sketch "Sketch6" against normal blind 4.315 contours L66 L68 A0 | A0 L67 L66 | A0 L65 L67 | L68 L65 A0 bodies 2
pattern_linear "Rectangular Pattern1" count 2 spacing 3.9624 along (0, 0, 1) count 12 spacing 2.54 along (-1, 0, 0) of "Extrusion3" bodies 2
equation "\"d29\" = pin_pitch"
equation "\"d32\" = row_pitch"
equation "\"d36\" = pin_offset"
equation "\"d41\" = pin_dia"
equation "\"d44\" = pin_pitch"
equation "\"d47\" = row_pitch"
equation "\"d54\" = row_pitch"
equation "\"d57\" = pin_pitch"
